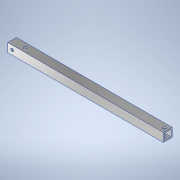
# Autodesk Inventor part: ハンド9x9_6
Saved by Autodesk Inventor 2020.3 (Build 243373000, 373)
## iProperties
Created: 2020-06-01
Part Number: ハンド9x9_6
Material: アルミニウム 6061
Document SubType Name: Modeling
Designer: totot
Density: 2.7 g/cm^3
Appearance: アルミニウム - フラット
Mass: 14.5203 g
Surface Area: 91.0592 cm^2
Volume: 5.37791 cm^3
Author: totot
Autodesk Inventor part; units mm, degrees
ref_plane "YZ Plane" through (0, 0, 0) normal (1, 0, 0) x (0, 1, 0)
ref_plane "XZ Plane" through (0, 0, 0) normal (0, 1, 0) x (-1, 0, 0)
ref_plane "XY Plane" through (0, 0, 0) normal (0, 0, 1) x (1, 0, 0)
sketch "スケッチ1" plane through (0, 0, 0) normal (1, 0, 0) x (0, 1, 0)
  line L0 (0, 0) -> (-9, 0)
  line L1 (-9, 0) -> (-9, -9)
  line L2 (-9, -9) -> (0, -9)
  line L3 (0, -9) -> (0, 0)
  line L4 (-1.2, -1.2) -> (-7.8, -1.2)
  line L5 (-7.8, -1.2) -> (-7.8, -7.8)
  line L6 (-7.8, -7.8) -> (-1.2, -7.8)
  line L7 (-1.2, -7.8) -> (-1.2, -1.2)
  dimension "d0" = 9
  dimension "d1" = 9
  dimension "d2" = 6.6
  dimension "d3" = 6.6
  dimension "d4" = 1.2
  dimension "d5" = 1.2
  constraints: 16 end point, 4 parallel, 2 horizontal, 2 perpendicular
  measures "d0" distance of L2.end L1.end
  measures "d1" distance of L1.end L0.end
  measures "d2" distance of L6.end L5.end
  measures "d3" distance of L6.end L4.start
  measures "d4" distance between parallel lines of L6 L2
  measures "d5" distance between parallel lines of L7 L3
extrude "押し出し1" add sketch "スケッチ1" along normal blind 145
sketch "スケッチ2" plane through (0, 0, 0) normal (0, 1, 0) x (1, 0, 0)
  line L0 (0, 9) -> (145, 9) projected
  line L1 (0, 9) -> (0, 0) projected
  line L2 (145, 9) -> (145, 0) projected
  point P0 (13.5, 4.5)
  point P1 (141.5, 4.5)
  dimension "d8" = 4.5
  dimension "d9" = 4.5
  dimension "d10" = 13.5
  dimension "d11" = 3.5
  measures "d8" distance from line of L0 point (141.5, 4.5)
  measures "d9" distance from line of point (13.5, 4.5) L0
  measures "d10" distance from line of point (13.5, 4.5) L1
  measures "d11" distance from line of point (141.5, 4.5) L2
hole "穴1" at (13.5, 0, -4.5) at (141.5, 0, -4.5) direction (0, -1, 0) diameter 3 end through all
sketch "スケッチ3" plane through (0, -9, 0) normal (0, 0, 1) x (1, 0, 0)
  line L0 (0, 9) -> (145, 9) projected
  line L1 (0, 9) -> (0, 0) projected
  point P0 (4.5, 4.5)
  dimension "d19" = 4.5
  dimension "d20" = 4.5
  measures "d19" distance from line of point (4.5, 4.5) L0
  measures "d20" distance from line of point (4.5, 4.5) L1
hole "穴2" at (4.5, -4.5, 0) direction (0, 0, -1) diameter 3 end through all
equation "\"d3\" = d2"
equation "\"d5\" = d4"
equation "\"d20\" = d19"
